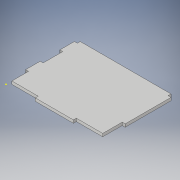
# Autodesk Inventor part: top_left_v2
Saved by Autodesk Inventor 2017.2 (Build 212233000, 233)
## iProperties
Created: 2017-06-09
Part Number: top_left_v2
Material: Generic
Document SubType Name: Modeling
Designer: SandeepSH
Density: 1 g/cm^3
Appearance: Default
Author: SandeepSH
Autodesk Inventor part; units mm, degrees
ref_plane "YZ Plane" through (0, 0, 0) normal (1, 0, 0) x (0, 1, 0)
ref_plane "XZ Plane" through (0, 0, 0) normal (0, 1, 0) x (-1, 0, 0)
ref_plane "XY Plane" through (0, 0, 0) normal (0, 0, 1) x (1, 0, 0)
sketch "Sketch1" plane through (0, 0, 0) normal (0, 1, 0) x (-1, 0, 0)
  point P0 (0, 0)
sketch "Sketch2" plane through (0, 0, 0) normal (0, 1, 0) x (-1, 0, 0)
  line L0 (0, 0) -> (-99, 0)
  line L1 (-99, 0) -> (-99, -90)
  line L2 (-99, -90) -> (0, -90)
  line L3 (0, -90) -> (0, 0)
  dimension "d0" = 99
  dimension "d1" = 90
  constraints: 8 end point, 2 parallel, 1 horizontal, 1 perpendicular
  measures "d0" distance of L2.end L1.end
  measures "d1" distance of L1.end L0.end
extrude "Extrusion1" add sketch "Sketch2" along normal blind 3
sketch "Sketch3" plane through (0, 3, 0) normal (0, 1, 0) x (1, 0, 0)
  line L0 (99, 0) -> (99, 90) projected
  line L1 (99, 0) -> (69, 0)
  line L2 (69, 0) -> (69, 3)
  line L3 (69, 3) -> (99, 3)
  line L4 (99, 3) -> (99, 0)
  line L5 (0, 0) -> (99, 0) projected
  line L6 (0, 0) -> (30, 0)
  line L7 (30, 0) -> (30, 3)
  line L8 (30, 3) -> (0, 3)
  line L9 (0, 3) -> (0, 0)
  line L10 (0, 3) -> (3, 3)
  line L11 (3, 3) -> (3, 20)
  line L12 (3, 20) -> (0, 20)
  line L13 (0, 20) -> (0, 3)
  line L14 (0, 90) -> (0, 0) projected
  line L15 (99, 3) -> (96, 3)
  line L16 (96, 3) -> (96, 23)
  line L17 (96, 23) -> (99, 23)
  line L18 (99, 23) -> (99, 3)
  line L19 (99, 90) -> (96, 90)
  line L20 (96, 90) -> (96, 70)
  line L21 (96, 70) -> (99, 70)
  line L22 (99, 70) -> (99, 90)
  line L23 (3, 35) -> (0, 35)
  line L24 (0, 35) -> (0, 55)
  line L25 (0, 55) -> (3, 55)
  line L26 (3, 55) -> (3, 35)
  line L27 (99, 90) -> (0, 90) projected
  line L28 (0, 90) -> (3, 90)
  line L29 (3, 90) -> (3, 70)
  line L30 (3, 70) -> (0, 70)
  line L31 (0, 70) -> (0, 90)
  dimension "d4" = 30
  dimension "d5" = 3
  dimension "d6" = 30
  dimension "d7" = 3
  dimension "d8" = 3
  dimension "d9" = 17
  dimension "d12" = 3
  dimension "d13" = 20
  dimension "d14" = 3
  dimension "d15" = 20
  dimension "d16" = 20
  dimension "d17" = 3
  dimension "d18" = 15
  dimension "d19" = 3
  dimension "d20" = 15
  constraints: 56 end point, 14 parallel, 7 horizontal, 7 perpendicular, 1 point on line
  measures "d4" distance of L2.end L3.end
  measures "d5" distance of L1.end L2.end
  measures "d6" distance of L8.end L7.end
  measures "d7" distance of L7.end L6.end
  measures "d8" distance of L12.end L11.end
  measures "d9" distance of L11.end L10.end
  measures "d12" distance of L16.end L17.end
  measures "d13" distance of L15.end L16.end
  measures "d14" distance of L21.end L20.end
  measures "d15" distance of L20.end L19.end
  measures "d16" distance of L23.end L24.end
  measures "d17" distance between parallel lines of L26 L14
  measures "d18" distance between parallel lines of L23 L12
  measures "d19" distance of L29.end L30.end
  measures "d20" distance between parallel lines of L30 L25
extrude "Extrusion2" cut sketch "Sketch3" against normal through all contours L1 L2 L3 L0 | L3 L16 L17 L0 | L5 L9 L8 L7 | L21 L20 L19 L0 | L13 L12 L11 L8 | L29 L30 L14 L27 | L14 L25 L26 L23
sketch "Sketch4" plane through (0, 3, 0) normal (0, 1, 0) x (1, 0, 0)
  line L0 (77.6899, 73) -> (37.1359, 73)
  line L1 (69, 3) -> (96, 3) projected
  line L2 (96, 90) -> (3, 90) projected
  line L3 (3, 90) -> (3, 70) projected
  line L4 (96, 90) -> (3, 90)
  line L5 (3, 90) -> (3, 73)
  line L6 (3, 73) -> (96, 73)
  line L7 (96, 73) -> (96, 90)
  point P0 (0, 0)
  dimension "d23" = 70
  dimension "d24" = 70
  constraints: 10 end point, 2 horizontal, 2 parallel, 1 perpendicular, 1 point on line
  measures "d23" distance between parallel lines of L1 L0
  measures "d24" distance between parallel lines of L1 L6
extrude "Extrusion3" cut sketch "Sketch4" against normal through all
body "Solid1"
